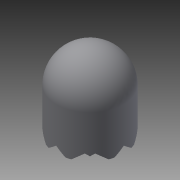
# Autodesk Inventor part: Ghost1
Saved by Autodesk Inventor 2015 (Build 190159000, 159)
## iProperties
Created: 2015-04-11
Part Number: Ghost1
Material: Generic
Document SubType Name: Modeling
Designer: tquinn
Density: 1 g/cm^3
Appearance: Default
Author: tquinn
Autodesk Inventor part; units mm, degrees
ref_plane "YZ Plane" through (0, 0, 0) normal (1, 0, 0) x (0, 1, 0)
ref_plane "XZ Plane" through (0, 0, 0) normal (0, 1, 0) x (-1, 0, 0)
ref_plane "XY Plane" through (0, 0, 0) normal (0, 0, 1) x (1, 0, 0)
sketch "Sketch1" plane through (0, 0, 0) normal (0, 0, 1) x (1, 0, 0)
  arc A0 (12.7, 3.175) -> (-12.7, 3.175) centre (0, 3.175) ccw
  line L0 (-12.7, 3.175) -> (-12.7, -12.7)
  line L1 (-12.7, -12.7) -> (12.7, -12.7)
  line L2 (12.7, -12.7) -> (12.7, 3.175)
  line L3 (-12.7, -12.7) -> (-11.1125, -12.7)
  line L4 (-11.1125, -12.7) -> (-7.9375, -12.7)
  line L5 (-7.9375, -12.7) -> (-7.9375, -10.16)
  line L6 (-7.9375, -10.16) -> (-11.1125, -12.7)
  line L7 (-7.9375, -10.16) -> (-4.7625, -12.7)
  line L8 (12.7, -12.7) -> (11.1125, -12.7)
  line L9 (11.1125, -12.7) -> (7.9375, -12.7)
  line L10 (7.9375, -12.7) -> (7.9375, -10.16)
  line L11 (7.9375, -10.16) -> (11.1125, -12.7)
  line L12 (7.9375, -12.7) -> (4.7625, -12.7)
  line L13 (4.7625, -12.7) -> (7.9375, -10.16)
  line L14 (0, -12.7) -> (0, -10.16)
  line L15 (0, -12.7) -> (3.175, -12.7)
  line L16 (3.175, -12.7) -> (0, -10.16)
  line L17 (0, -12.7) -> (-3.175, -12.7)
  line L18 (-3.175, -12.7) -> (0, -10.16)
  dimension "d5" = 25.4
  dimension "d6" = 15.875
  dimension "d7" = 25.4
  dimension "d8" = 1.5875
  dimension "d9" = 3.175
  dimension "d10" = 2.54
  dimension "d11" = 3.175
  dimension "d12" = 1.5875
  dimension "d13" = 3.175
  dimension "d14" = 2.54
  dimension "d15" = 3.175
  dimension "d16" = 2.54
  dimension "d17" = 3.175
  dimension "d18" = 3.175
  constraints: 36 end point, 4 vertical, 2 point on circle, 2 tangent, 1 centre point, 1 perpendicular, 12 other
  measures "d5" diameter of A0
  measures "d6" distance of L2.start L2.end
  measures "d7" distance of L0.end L2.start
  measures "d8" distance of L0.end L3.end
  measures "d9" distance of L3.end L4.end
  measures "d10" distance of L4.end L5.end
  measures "d11" distance from line of L7.end L5
  measures "d12" distance of L2.start L8.end
  measures "d13" distance of L8.end L9.end
  measures "d14" distance of L9.end L10.end
  measures "d15" distance of L9.end L12.end
  measures "d16" distance of L14.start L14.end
  measures "d17" distance of L14.start L15.end
  measures "d18" distance of L14.start L17.end
extrude "Extrusion1" add sketch "Sketch1" along normal blind 25.4 contours L2 L1 L11 L13 L16 L18 L7 L6 L0 A0
fillet "Fillet1" radius 12.7 6 edges at (-12.7, -4.7625, 25.4) (12.7, -4.7625, 25.4) (0, 15.875, 25.4) (-12.7, -4.7625, 0) (12.7, -4.7625, 0) (0, 15.875, 0)
sketch "Sketch2" plane through (0, 0, 0) normal (1, 0, 0) x (0, 1, 0)
  arc A0 (3.1749, 0) -> (3.1749, 25.4) centre (3.1749, 12.7) ccw
  line L0 (3.1749, 25.4) -> (-12.7001, 25.4)
  line L1 (-12.7001, 25.4) -> (-12.7001, 0)
  line L2 (-12.7001, 0) -> (3.1749, 0)
  line L3 (-12.7001, 25.4) -> (-12.7001, 23.8125)
  line L4 (-12.7001, 23.8125) -> (-12.7001, 20.6375)
  line L5 (-12.7001, 20.6375) -> (-10.1601, 20.6375)
  line L6 (-10.1601, 20.6375) -> (-12.7001, 23.8125)
  line L7 (-10.1601, 20.6375) -> (-12.7001, 17.4625)
  line L8 (-12.7001, 0) -> (-12.7001, 1.5875)
  line L9 (-12.7001, 1.5875) -> (-12.7001, 4.7625)
  line L10 (-12.7001, 4.7625) -> (-10.1601, 4.7625)
  line L11 (-10.1601, 4.7625) -> (-12.7001, 1.5875)
  line L12 (-12.7001, 4.7625) -> (-12.7001, 7.9375)
  line L13 (-12.7001, 7.9375) -> (-10.1601, 4.7625)
  line L14 (-12.7001, 12.7) -> (-10.1601, 12.7)
  line L15 (-12.7001, 12.7) -> (-12.7001, 9.525)
  line L16 (-12.7001, 9.525) -> (-10.1601, 12.7)
  line L17 (-12.7001, 12.7) -> (-12.7001, 15.875)
  line L18 (-12.7001, 15.875) -> (-10.1601, 12.7)
  line L19 (3.175, 25.4) -> (3.175, 0) projected
  point P0 (0, 0)
  dimension "d22" = 25.4
  dimension "d23" = 15.875
  dimension "d24" = 25.4
  dimension "d25" = 1.5875
  dimension "d26" = 3.175
  dimension "d27" = 2.54
  dimension "d28" = 3.175
  dimension "d29" = 1.5875
  dimension "d30" = 3.175
  dimension "d31" = 2.54
  dimension "d32" = 3.175
  dimension "d33" = 2.54
  dimension "d34" = 3.175
  dimension "d35" = 3.175
  constraints: 36 end point, 2 point on circle, 2 tangent, 1 centre point, 1 horizontal, 1 perpendicular, 12 other
  measures "d22" diameter of A0
  measures "d23" distance of L2.start L2.end
  measures "d24" distance of L0.end L2.start
  measures "d25" distance of L0.end L3.end
  measures "d26" distance of L3.end L4.end
  measures "d27" distance of L4.end L5.end
  measures "d28" distance from line of L7.end L5
  measures "d29" distance of L2.start L8.end
  measures "d30" distance of L8.end L9.end
  measures "d31" distance of L9.end L10.end
  measures "d32" distance of L9.end L12.end
  measures "d33" distance of L14.start L14.end
  measures "d34" distance of L14.start L15.end
  measures "d35" distance of L14.start L17.end
extrude "Extrusion2" cut sketch "Sketch2" along normal mid plane 25.4 contours L19 A0 | L2 L1 L11 L13 L16 L18 L7 L6 L0 L19 keep common part
equation "\"d6\" = 0.625 * d5"
equation "\"d7\" = d5"
equation "\"d8\" = 0.0625 * d7"
equation "\"d9\" = 0.125 * d7"
equation "\"d11\" = d9"
equation "\"d12\" = d8"
equation "\"d13\" = d9"
equation "\"d14\" = d10"
equation "\"d15\" = d9"
equation "\"d16\" = d10"
equation "\"d17\" = d9"
equation "\"d18\" = d9"
equation "\"d23\" = 0.625 * d22"
equation "\"d24\" = d22"
equation "\"d25\" = 0.0625 * d24"
equation "\"d26\" = 0.125 * d24"
equation "\"d28\" = d26"
equation "\"d29\" = d25"
equation "\"d30\" = d26"
equation "\"d31\" = d27"
equation "\"d32\" = d26"
equation "\"d33\" = d27"
equation "\"d34\" = d26"
equation "\"d35\" = d26"
body "Solid1"
